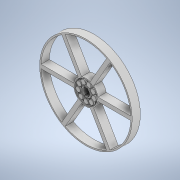
# Autodesk Inventor part: PIP-KL_parametriserad_02
Saved by Autodesk Inventor 2021 (Build 250183000, 183)
## iProperties
Created: 2020-11-21
Part Number: PIP-KL_parametriserad_02
Material: Generic
Document SubType Name: Modeling
Designer: Gottfrid
Density: 1 g/cm^3
Appearance: Default
d_inreRing: 2.500 mm
d_yttreRing: 2.500 mm
r_yttre: 10.000 mm
h_rullager: 7,500 mm
Author: Gottfrid
Autodesk Inventor part; units mm, degrees
ref_plane "YZ Plane" through (0, 0, 0) normal (1, 0, 0) x (0, 1, 0)
ref_plane "XZ Plane" through (0, 0, 0) normal (0, 1, 0) x (-1, 0, 0)
ref_plane "XY Plane" through (0, 0, 0) normal (0, 0, 1) x (1, 0, 0)
sketch "Sketch1" plane through (0, 0, 0) normal (0, 0, 1) x (1, 0, 0)
  circle A0 centre (0, 0) radius 3.5
  circle A1 centre (0, 0) radius 4.75
  circle A2 centre (0, 0) radius 10
  circle A3 centre (0, 0) radius 11.25
  circle A4 centre (0, -7.375) radius 2.375
  line L0 (1.2333, -3.7857) -> (-1.2333, -3.7857)
  line L1 (-1.6333, -3.3857) -> (-1.6333, 3.3857)
  line L2 (-1.2333, 3.7857) -> (1.2333, 3.7857)
  line L3 (1.6333, 3.3857) -> (1.6333, -3.3857)
  line L4 (1.6333, -3.7857) -> (-1.6333, 3.7857) construction
  line L5 (-1.6333, -3.7857) -> (1.6333, 3.7857) construction
  arc A5 (-1.2333, 3.7857) -> (-1.6333, 3.3857) centre (-1.2333, 3.3857) ccw
  arc A6 (1.6333, 3.3857) -> (1.2333, 3.7857) centre (1.2333, 3.3857) ccw
  arc A7 (1.2333, -3.7857) -> (1.6333, -3.3857) centre (1.2333, -3.3857) ccw
  arc A8 (-1.6333, -3.3857) -> (-1.2333, -3.7857) centre (-1.2333, -3.3857) ccw
  circle A9 centre (0, 0) radius 42.5
  circle A10 centre (0, 0) radius 41.25
  line L6 (11.1051, 1.8) -> (41.2107, 1.8)
  line L7 (-59.5, 0) -> (59.5, 0) projected
  line L8 (11.1051, -1.8) -> (41.2107, -1.8)
  line L9 (3.9937, 10.5173) -> (19.0465, 36.5895)
  line L10 (7.1114, 8.7173) -> (22.1642, 34.7895)
  line L11 (-7.1114, 8.7173) -> (-22.1642, 34.7895)
  line L12 (-3.9937, 10.5173) -> (-19.0465, 36.5895)
  line L13 (-11.1051, -1.8) -> (-41.2107, -1.8)
  line L14 (-11.1051, 1.8) -> (-41.2107, 1.8)
  line L15 (-3.9937, -10.5173) -> (-19.0465, -36.5895)
  line L16 (-7.1114, -8.7173) -> (-22.1642, -34.7895)
  line L17 (7.1114, -8.7173) -> (22.1642, -34.7895)
  line L18 (3.9937, -10.5173) -> (19.0465, -36.5895)
  point P0 (-1.6333, 3.0955)
  point P1 (1.6333, 3.0955)
  point P2 (1.6333, -3.0955)
  point P3 (-1.6333, -3.0955)
  point P4 (-19.0465, 36.5895)
  dimension "d3" = 22.5
  dimension "d83" = 82.5
  dimension "d0" = 7
  dimension "d1" = 9.5
  dimension "d2" = 20
  dimension "d4" = 7.375
  dimension "d5" = 4.75
  dimension "d64" = 7.5714
  dimension "d65" = 3.2667
  dimension "d66" = 0.4
  dimension "d82" = 85
  dimension "d85" = 1.8
  dimension "d88" = 360
  constraints: 36 end point, 9 centre point, 8 point on circle, 8 point on line, 8 tangent, 6 coincident, 3 equal radius, 2 horizontal, 2 midpoint, 2 parallel, 2 symmetric about line, 1 perpendicular, 1 vertical alignment, 43 other
  measures "d0" diameter of A0
  measures "d1" diameter of A1
  measures "d2" diameter of A2
  measures "d4" distance of A4.centre point (0, 0)
  measures "d5" diameter of A4
  measures "d64" distance between parallel lines of L0 L2
  measures "d65" distance between parallel lines of L3 L1
  measures "d66" radius of A5
  measures "d82" diameter of A9
  measures "d85" distance between parallel lines of L7 L6
extrude "Extrusion1" add sketch "Sketch1" along normal blind 1.5 contours L7 L3 A0 | L7 A1 A0 L1 A8 L0 A7 L3 | A0 L3 A6 L2 A5 L1 L7 A1 | A0 L3 L7 | L3 L7 L1 A0 | A0 L1 A5 L2 A6 L3 | L3 A7 L0 A8 L1 A0 | A0 L1 L7 L3 | L1 L7 A0 | A0 L7 L1
extrude "Extrusion8" add sketch "Sketch1" along normal blind 1.5 contours A4
extrude "Extrusion9" add sketch "Sketch1" along normal blind 1.5 contours L7 A3 A2 | A2 L7 A3
sketch "Sketch17" plane through (0, 0, 1.5) normal (0, 0, 1) x (1, 0, 0)
  circle A0 centre (0, 0) radius 4.75 projected
extrude "Extrusion10" add sketch "Sketch17" along normal blind 1.5 draft 35
sketch "Sketch18" plane through (0, -7.375, 1.5) normal (0, 0, 1) x (1, 0, 0)
  circle A0 centre (0, 0) radius 2.375 projected
  point P0 (0, 7.375)
extrude "Extrusion11" add sketch "Sketch18" along normal blind 1.5 draft -35
sketch "Sketch19" plane through (0, 0, 1.5) normal (0, 0, 1) x (1, 0, 0)
  circle A0 centre (0, 0) radius 10 projected
  circle A1 centre (0, 0) radius 11.25 projected
extrude "Extrusion12" add sketch "Sketch19" along normal blind 1.5 draft 35
sketch "Sketch20" plane through (0, 0, 3) normal (0, 0, 1) x (1, 0, 0)
  circle A0 centre (0, 0) radius 5.8003 projected
extrude "Extrusion13" add sketch "Sketch20" along normal blind 0.75
sketch "Sketch21" plane through (0, -7.375, 3) normal (0, 0, 1) x (1, 0, 0)
  circle A0 centre (0, 0) radius 1.3247 projected
  point P0 (0, 7.375)
extrude "Extrusion14" add sketch "Sketch21" along normal blind 0.75
sketch "Sketch22" plane through (0, 0, 3) normal (0, 0, 1) x (1, 0, 0)
  circle A0 centre (0, 0) radius 8.9497 projected
  circle A1 centre (0, 0) radius 12.3003 projected
extrude "Extrusion15" add sketch "Sketch22" along normal blind 0.75
chamfer "Chamfer6" distance 0.3 angle 45 1 edges at (-10, 0, 0)
chamfer "Chamfer2" distance 0.3 angle 45 1 edges at (-2.375, -7.375, 0)
chamfer "Chamfer5" distance 0.3 angle 45 1 edges at (-4.75, 0, 0)
mirror "Mirror1" about plane through (0, 0, 3.75) normal (0, 0, 1) of "Extrusion13", "Extrusion10", "Extrusion1", "Chamfer5"
mirror "Mirror2" about plane through (0, -7.375, 3.75) normal (0, 0, 1) of "Extrusion8", "Extrusion11", "Extrusion14", "Chamfer2"
mirror "Mirror3" about plane through (0, 0, 3.75) normal (0, 0, 1) of "Extrusion9", "Extrusion12", "Extrusion15", "Chamfer6"
extrude "Extrusion18" cut sketch "Sketch1" along normal blind 999 contours A0 L1 A5 L2 A6 L3 | L3 A7 L0 A8 L1 A0
pattern_circular "Circular Pattern3" count 9 over 360 about axis through (0, 0, -10) along (0, 0, 1) of "Extrusion8", "Extrusion11", "Extrusion14", "Chamfer2", "Mirror2"
extrude "Extrusion19" cut sketch "Sketch1" along normal blind 999 contours L7 L3 A0 | A0 L3 L7 | L3 L7 L1 A0 | A0 L1 L7 L3 | L1 L7 A0 | A0 L7 L1
extrude "Extrusion20" cut sketch "Sketch1" along normal blind 999 contours L7 L3 A0 | L7 A1 A0 L1 A8 L0 A7 L3 | A0 L3 A6 L2 A5 L1 L7 A1 | A0 L3 L7 | L3 L7 L1 A0 | A0 L1 A5 L2 A6 L3 | L3 A7 L0 A8 L1 A0 | A0 L1 L7 L3 | L7 A2 A1 | A1 L7 A2 | L1 L7 A0 | A0 L7 L1 | L7 A3 A2 | A2 L7 A3 | A4 keep common part
extrude "Extrusion21" add sketch "Sketch1" along normal blind 7.5 contours L7 A10 L8 A3 | A3 L6 A10 L7 | L7 A10 L14 A3 | A3 L13 A10 L7 | L7 A9 A10 | A10 L7 A9 | A3 L9 A10 L10 | L17 A10 L18 A3 | L11 A10 L12 A3 | A3 L15 A10 L16
equation "\"d3\" = 2 * r_yttre + d_yttreRing"
equation "\"d83\" = D_yttreSpolRotor - d_yttreRing"
equation "\"d0\" = D_axel"
equation "\"d1\" = D_axel + d_inreRing"
equation "\"d2\" = 2 * r_yttre"
equation "\"d4\" = beräknad_avstånd_origo_till_rullkopp"
equation "\"d5\" = beräknad_diameter_rullkropp"
equation "\"d66\" = r_filletAxel"
equation "\"d82\" = D_yttreSpolRotor"
equation "\"d85\" = d_stöttor"
equation "\"d6\" = extrude_h1"
equation "\"d29\" = extrude_h1"
equation "\"d31\" = extrude_h1"
equation "\"d33\" = extrude_h1"
equation "\"d34\" = extrude_angle35"
equation "\"d35\" = extrude_h1"
equation "\"d36\" = -extrude_angle35"
equation "\"d37\" = extrude_h1"
equation "\"d38\" = extrude_angle35"
equation "\"d39\" = 0.5 * extrude_h1"
equation "\"d41\" = 0.5 * extrude_h1"
equation "\"d43\" = 0.5 * extrude_h1"
equation "\"d72\" = 0.2 * extrude_h1"
equation "\"d45\" = 0.2 * extrude_h1"
equation "\"d69\" = 0.2 * extrude_h1"
equation "\"r_inre\" = 0.5 * D_axel"
equation "\"d_inreRing\" = 2.5"
equation "\"r_yttre\" = 10"
equation "\"d_yttreRing\" = 2.5"
equation "\"d_toleransMellanRullkroppOchRing\" = 0.25"
equation "\"extrude_h1\" = 0.2 * h_rullager"
equation "\"extrude_angle35\" = 35deg"
equation "\"beräknad_diameter_rullkropp\" = r_yttre - 0.5 * d_inreRing - r_inre - 2 * d_toleransMellanRullkroppOchRing"
equation "\"beräknad_avstånd_origo_till_rullkopp\" = 0.5 * d_inreRing + r_inre + 0.5 * beräknad_diameter_rullkropp + d_toleransMellanRullkroppOchRing"
equation "\"D_axel\" = 7"
equation "\"d_axelRing\" = 3"
equation "\"r_filletAxel\" = 0.4"
equation "\"h_rullager\" = 7.5"
equation "\"D_yttreSpolRotor\" = 85"
equation "\"d_stöttor\" = 1.8"
body "Solid1"
